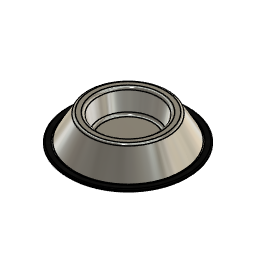
day11-dog_bowl (Autodesk Fusion 360 design; units mm, degrees)
part number: 2025-06-24-21-06-45-082
Autodesk Fusion 360 part; units mm, degrees
sketch "Sketch1" plane through (0, 0, 0) normal (0, 1, 0) x (1, 0, 0)
  line L0 (0, 0) -> (110, 0) construction
  line L1 (110, 0) -> (110, -2.5)
  line L2 (110, -2.5) -> (100, -2.5)
  line L3 (100, -2.5) -> (72.5, -50.1314)
  line L4 (72.5, -50.1314) -> (57.5, -50.1314)
  line L5 (0, -10) -> (50.4238, -10)
  line L6 (57.5, -50.1314) -> (50.4238, -10)
  line L7 (48.6605, 0) -> (48.646, 0.082)
  dimension "d1" = 110
  dimension "d2" = 2.5
  dimension "d3" = 10
  dimension "d4" = 120
  dimension "d5" = 55
  dimension "d6" = 15
  dimension "d7" = 10
  dimension "d8" = 100
  constraint coincident L0.start origin
  constraint horizontal L0
  constraint perpendicular L0 L1
  constraint perpendicular L1 L2
  constraint parallel L0 L4
  constraint horizontal L5
  constraint coincident L0 L7.start
  constraint collinear L6 L7
  constraint vertical L0.start L5.start
  measures "d1" distance of L0.start L0.end
  measures "d2" distance of L0.end L1.end
  measures "d3" distance of L1.end L2.end
  measures "d4" angle of L2 L3
  measures "d5" distance of L2.end L3.end
  measures "d6" distance of L3.end L4.end
  measures "d7" distance of L0 L5
  measures "d8" angle of L5 L6
surface "Revolve2" add revolved angle 360 about axis through (0, 0, 1.75) along (0, 0, 20.75) path "Sketch1" along L1 L2 L3 L4 L6 L5 makes body 1
fillet "Fillet3" radius 5 3 edges at (-53.6088, -20.7929, 50.1314) (-67.5937, -26.2171, 50.1314) (-47.0114, -18.234, 10) on bodies 1
fillet "Fillet3" radius 2.5 1 edges at (-93.2327, -36.1615, 2.5) on bodies 1
thicken "Thicken1" add thickness -2.5 9 faces at (-33.1851, -84.5544, 18.3771) (-8.8696, -70.7774, 49.8271) (66.4851, -6.5235, 50.1314) (57.7562, 21.0215, 50.126) (49.4618, -23.8195, 35.377) (49.3323, 12.5616, 13.2353) (-22.0551, 13.7998, 10) (87.4079, -47.5998, 3.393) (106.3606, -10.5047, 2.5) separate body on bodies 1 makes body 2
fillet "Fillet4" radius 0.5 1 edges at (-102.556, -39.7777, 2.5) on bodies 2
fillet "Fillet5" radius 0.5 1 edges at (-102.556, -39.7777, 0) on bodies 2
offset_surface "SurfaceOffset1" offset 0.3 5 faces at (106.4068, -5.44, 0) (87.6312, 66.378, 0.25) (19.1013, -108.3289, 1) (-13.6695, -109.0798, 2.25) (106.4068, -5.44, 2.5) on bodies 2 makes body 3
thicken "Thicken2" add thickness 1 5 faces at (106.4068, -5.44, 2.8) (50.2711, -98.0575, 2.4) (-29.8737, -106.1775, 1) (87.8383, 66.5349, 0.1) (106.4068, -5.44, -0.3) separate body on bodies 3 makes body 4
hidden bodies 1 3
